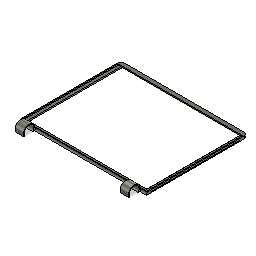
B_case (Autodesk Fusion 360 design; units mm, degrees)
Autodesk Fusion 360 part; units mm, degrees
note: some values were not read from the file. Set by a fixed rule: which sketch regions a step uses.
sketch "Sketch1" plane through (0, 0, 0) normal (0, 1, 0) x (1, 0, 0)
  line L0 (0, 0) -> (230.6, 0)
  line L1 (230.6, 0) -> (230.6, 183)
  line L2 (230.6, 183) -> (0, 183)
  line L3 (0, 183) -> (0, 0)
  dimension "d1" = 230.6
  dimension "d2" = 183
  constraint horizontal L0
  constraint vertical L1
  constraint horizontal L2
  constraint vertical L3
  constraint coincident L0.start L3.end
  measures "d1" distance of L0.start L0.end
  measures "d2" distance of L0.start L2.end
extrude "Extrude1" add sketch "Sketch1" along normal blind 10
sketch "Sketch9" plane through (0, 0, 0) normal (-1, 0, 0) x (0, 0, 1)
  line L0 (-183, 0) -> (0, 0)
  line L1 (0, 0) -> (0, 10)
  line L2 (0, 10) -> (-183, 10)
  line L3 (-183, 10) -> (-183, 0)
  circle A0 centre (11.4881, 10.5) radius 10.5
  line L4 (11.4881, 0) -> (0, 0)
  circle A1 centre (11.4881, 10.5) radius 9
  line L5 (0, 0) -> (1, 0)
  line L6 (1, 0) -> (1, 10)
  line L7 (1, 10) -> (0, 10)
  line L8 (0, 10) -> (0, 0)
  dimension "d69" = 21
  dimension "d70" = 18
  dimension "d94" = 1
  constraint coincident A0 L4.start
  constraint coincident L0.end L1.start
  constraint tangent A0 L4
  constraint parallel L0 L4
  constraint concentric A0 A1
  constraint horizontal L5
  constraint vertical L6
  constraint horizontal L7
  constraint vertical L8
  constraint coincident A0 L6.end
  constraint collinear L2 L7
  measures "d69" diameter of A0
  measures "d70" diameter of A1
  measures "d94" distance of L0.end L5.end
extrude "Extrude8" add sketch "Sketch9" against normal up to surface (230.6 mm away) contours L1 L4 L5 L6 L7 L8 | A0 L4 L6 | A0
sketch "Sketch10" plane through (0, 0, 0) normal (0, -1, 0) x (1, 0, 0)
  line L0 (230.6, -183) -> (230.6, 11.4881)
  line L1 (230.6, 11.4881) -> (0, 11.4881)
  line L2 (0, 11.4881) -> (0, -183)
  line L3 (230.6, 0) -> (218.6, 0)
  line L4 (218.6, 0) -> (218.6, 22)
  line L5 (218.6, 22) -> (230.6, 22)
  line L6 (230.6, 22) -> (230.6, 0)
  line L7 (203.6, 0) -> (27, 0)
  line L8 (27, 0) -> (27, 22)
  line L9 (27, 22) -> (203.6, 22)
  line L10 (203.6, 22) -> (203.6, 0)
  line L11 (0, 0) -> (12, 0)
  line L12 (12, 0) -> (12, 22)
  line L13 (12, 22) -> (0, 22)
  line L14 (0, 22) -> (0, 0)
  line L15 (0, -183) -> (230.6, -183)
  dimension "d73" = 22
  dimension "d74" = 12
  dimension "d75" = 12
  dimension "d76" = 15
  dimension "d77" = 15
  constraint vertical L4
  constraint horizontal L5
  constraint vertical L6
  constraint horizontal L7
  constraint vertical L8
  constraint horizontal L9
  constraint vertical L10
  constraint horizontal L11
  constraint vertical L12
  constraint horizontal L13
  constraint vertical L14
  constraint coincident L11.start L14.end
  constraint collinear L5 L9
  constraint collinear L9 L13
  constraint collinear L0 L6
  constraint parallel L1 L3
  constraint collinear L3 L7
  constraint collinear L7 L11
  measures "d73" distance of L3.start L5.end
  measures "d74" distance of L3.start L3.end
  measures "d75" distance of L12.end L13.end
  measures "d76" distance of L8 L12
  measures "d77" distance of L4 L10
extrude "Extrude9" cut sketch "Sketch10" against normal through all contours L0 L1 L3 L4 L6 | L1 L4 L5 L6 | L1 L2 L11 L12 L14 | L1 L12 L13 L14 | L1 L7 L8 L10 | L1 L8 L9 L10
sketch "Sketch11" plane through (0, 10, 0) normal (0, 1, 0) x (-1, 0, 0)
  line L0 (0, -183) -> (0, 0)
  line L1 (-1.8, -176) -> (-228.8, -176)
  line L2 (-228.8, -176) -> (-228.8, -1)
  line L3 (-228.8, -1) -> (-1.8, -1)
  line L4 (-1.8, -1) -> (-1.8, -176)
  line L5 (-115.3, -124.4699) -> (-115.3, -51.5615) construction
  line L6 (-230.6, 0) -> (-230.6, -183)
  line L7 (-230.6, -183) -> (0, -183)
  line L8 (-12, 0) -> (-12, 1)
  line L9 (-12, 1) -> (-27, 1)
  line L10 (-27, 1) -> (-27, 0)
  line L11 (-27, 0) -> (-203.6, 0)
  line L12 (-203.6, 0) -> (-203.6, 1)
  line L13 (-203.6, 1) -> (-218.6, 1)
  line L14 (-218.6, 1) -> (-218.6, 0)
  line L15 (-218.6, 0) -> (-230.6, 0)
  line L16 (0, 0) -> (-12, 0)
  dimension "d79" = 227
  dimension "d80" = 175
  dimension "d100" = 1
  constraint horizontal L1
  constraint vertical L2
  constraint horizontal L3
  constraint vertical L4
  constraint symmetric L2 L4 L5
  constraint symmetric L0 L5 L6
  measures "d79" distance of L1.start L1.end
  measures "d80" distance of L1.start L3.end
  measures "d100" distance of L3 L16
extrude "Extrude10" cut sketch "Sketch11" against normal blind 2 contours L1 L2 L3 L4
sketch "Sketch12" plane through (0, 8, 0) normal (0, 1, 0) x (-1, 0, 0)
  line L0 (-1.8, -1) -> (-228.8, -1)
  line L1 (-1.8, -176) -> (-1.8, -1)
  line L2 (-6.95, -6.345) -> (-223.65, -6.345)
  line L3 (-223.65, -6.345) -> (-223.65, -182.345)
  line L4 (-223.65, -182.345) -> (-6.95, -182.345)
  line L5 (-6.95, -182.345) -> (-6.95, -6.345)
  line L6 (-10.47, -167.125) -> (-220.13, -167.125)
  line L7 (-220.13, -167.125) -> (-220.13, -9.875)
  line L8 (-220.13, -9.875) -> (-10.47, -9.875)
  line L9 (-10.47, -9.875) -> (-10.47, -167.125)
  line L10 (-83.8338, -88.5) -> (-143.8338, -88.5) construction
  line L11 (-115.3, -111.7944) -> (-115.3, -61.4121) construction
  line L12 (-228.8, -1) -> (-228.8, -176)
  line L13 (-228.8, -176) -> (-1.8, -176)
  dimension "d84" = 176
  dimension "d85" = 216.7
  dimension "d86" = 209.66
  dimension "d87" = 157.25
  dimension "d88" = 3.52
  dimension "d89" = 3.53
  constraint horizontal L2
  constraint vertical L3
  constraint horizontal L4
  constraint vertical L5
  constraint horizontal L6
  constraint vertical L7
  constraint horizontal L8
  constraint vertical L9
  constraint parallel L3 L11
  constraint symmetric L7 L9 L11
  constraint symmetric L6 L8 L10
  constraint symmetric L0 L10 L13
  constraint symmetric L1 L11 L12
  measures "d84" distance of L2.start L4.end
  measures "d85" distance of L3.end L4.end
  measures "d86" distance of L6.start L6.end
  measures "d87" distance of L6.start L8.end
  measures "d88" distance of L5 L9
  measures "d89" distance of L2 L8
extrude "Extrude11" cut sketch "Sketch12" against normal blind 2.6 contours L2 L3 L5 L13 | L3 L4 L5 L13 | L6 L7 L8 L9
fillet "Fillet1" radius 6 2 edges at (0, 5, -183) (230.6, 5, -183)
sketch "Sketch15" plane through (12, 0, 0) normal (-1, 0, 0) x (0, 0, 1)
  line L0 (1, 10) -> (0, 10)
  line L1 (0, 10) -> (0, 0)
  line L2 (0, 0) -> (11.4881, 0)
  arc A0 (11.4881, 0) -> (1, 10) centre (11.4881, 10.5) ccw
  circle A1 centre (11.4881, 10.5) radius 9
  circle A2 centre (11.4881, 10.5) radius 11.499
  line L3 (0, 0) -> (6.8002, 0)
  constraint concentric A0 A2
  constraint coincident L0.end A2
  constraint coincident L1.end L2.start
  constraint coincident L2 L3.end
  constraint coincident A2 L3.end
extrude "Extrude14" add sketch "Sketch15" along normal blind 12 and the other way blind 218.6 contours L1 L2 A2 L3
sketch "Sketch13" plane through (0, 0, 0) normal (-1, 0, 0) x (0, 0, 1)
  line L0 (-177, 10) -> (-177, 0)
  line L1 (-177, 0) -> (6.8002, 0)
  line L2 (0, 10) -> (-177, 10)
  line L3 (-187, -4.6) -> (23, -4.6)
  line L4 (23, -4.6) -> (23, 5.4)
  line L5 (23, 5.4) -> (-187, 5.4)
  line L6 (-187, 5.4) -> (-187, -4.6)
  arc A0 (0, 10) -> (6.8002, 0) centre (11.4881, 10.5) ccw
  dimension "d95" = 4.6
  dimension "d96" = 10
  dimension "d97" = 10
  dimension "d98" = 210
  constraint horizontal L3
  constraint vertical L4
  constraint horizontal L5
  constraint vertical L6
  measures "d95" distance of L2 L5
  measures "d96" distance of L3.start L5.end
  measures "d97" distance of L0 L6
  measures "d98" distance of L3.start L3.end
extrude "Extrude12" cut sketch "Sketch13" against normal through all contours L0 L1 L5 A0 | L0 L1 L3 L4 L5 L6 A0
sketch "Sketch14" plane through (0, 5.4, 0) normal (0, -1, 0) x (1, 0, 0)
  line L0 (218.6, 18.9036) -> (218.6, 20.6663)
  line L1 (12, 18.9036) -> (27, 18.9036)
  line L2 (203.6, 20.6663) -> (203.6, 18.9036)
  line L3 (27, 18.9036) -> (27, 20.6663)
  line L4 (12, 20.6663) -> (12, 18.9036)
  line L5 (27, 20.6663) -> (12, 20.6663)
  line L6 (203.6, 18.9036) -> (218.6, 18.9036)
  line L7 (218.6, 20.6663) -> (203.6, 20.6663)
  line L8 (223.65, -8.545) -> (230.45, -8.545)
  line L9 (230.45, -8.545) -> (230.45, -168.645)
  line L10 (230.45, -168.645) -> (223.65, -168.645)
  line L11 (223.65, -168.645) -> (223.65, -8.545)
  line L12 (223.65, -182.345) -> (223.65, -6.345)
  dimension "d101" = 6.8
  dimension "d102" = 2.2
  dimension "d103" = 160.1
  constraint horizontal L8
  constraint vertical L9
  constraint horizontal L10
  constraint vertical L11
  constraint collinear L11 L12
  measures "d101" distance of L9.end L10.end
  measures "d102" distance of L8 L12.end
  measures "d103" distance of L8.end L9.end
extrude "Extrude13" cut sketch "Sketch14" against normal blind 1.6 contours L8 L9 L10 L11 L12
